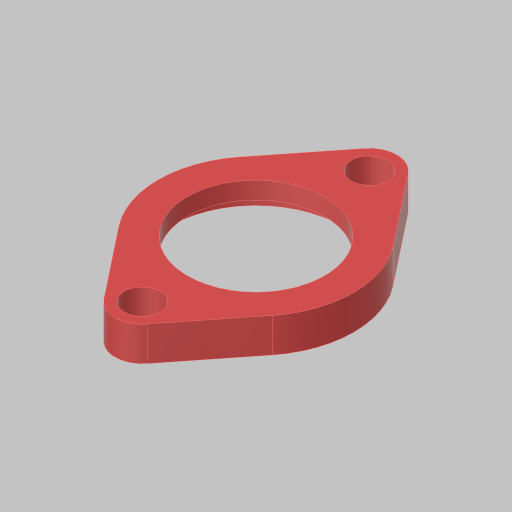
# Autodesk Inventor part: Retainer
Saved by Autodesk Inventor 2023.5 (Build 275446000, 446)
## iProperties
Created: 2025-01-25
Part Number: Retainer
Material: ABS Plastic
Document SubType Name: Modeling
Designer: slick
Density: 1.06 g/cm^3
Appearance: Smooth - Red
Author: slick
Autodesk Inventor part; units mm, degrees
ref_plane "YZ Plane" through (0, 0, 0) normal (1, 0, 0) x (0, 1, 0)
ref_plane "XZ Plane" through (0, 0, 0) normal (0, 1, 0) x (-1, 0, 0)
ref_plane "XY Plane" through (0, 0, 0) normal (0, 0, 1) x (1, 0, 0)
sketch "Sketch1" plane through (0, 0, 0) normal (0, 1, 0) x (-1, 0, 0)
  circle A0 centre (0, 0) radius 12.7
  circle A1 centre (0, 0) radius 18.0975
  circle A2 centre (0, 21.0185) radius 5.08 construction
  circle A3 centre (0, -21.0185) radius 5.08 construction
  line L0 (3.9884, 24.1647) -> (14.2088, 11.2084)
  line L1 (-3.9884, 24.1647) -> (-14.2088, 11.2084)
  line L2 (-14.2088, -11.2084) -> (-3.9884, -24.1647)
  line L3 (3.9884, -24.1647) -> (14.2088, -11.2084)
  arc A4 (14.2088, -11.2084) -> (14.2088, 11.2084) centre (0, 0) ccw
  arc A5 (-3.9884, -24.1647) -> (3.9884, -24.1647) centre (0, -21.0185) ccw
  arc A6 (-14.2088, 11.2084) -> (-14.2088, -11.2084) centre (0, 0) ccw
  arc A7 (3.9884, 24.1647) -> (-3.9884, 24.1647) centre (0, 21.0185) ccw
  circle A8 centre (0, 0) radius 15.9385
  dimension "d0" = 25.4
  dimension "d1" = 36.195
  dimension "d2" = 10.16
  dimension "d7" = 31.877
  dimension "d15" = 42.037
  constraints: 16 point on circle, 10 tangent, 9 centre point, 9 coincident, 8 end point, 3 equal radius, 2 vertical alignment
  measures "d0" diameter of A0
  measures "d1" diameter of A1
  measures "d2" diameter of A2
  measures "d7" diameter of A8
  measures "d15" distance of A7.centre A3.centre
extrude "Extrusion1" add sketch "Sketch1" along normal blind 6.35 contours A1 | A1 L1 A7 L0 | L3 A5 L2 A1 | A8
extrude "Extrusion2" cut sketch "Sketch1" along normal blind 3.175 contours A8
hole "Hole1" at (0, 0, 21.0185) at (0, 0, -21.0185) direction (0, 1, 0) diameter 6.7 end through all
body "Solid1"
